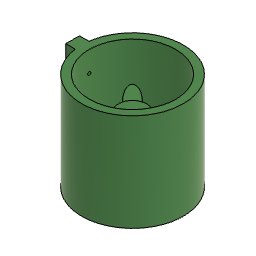
Propeller (Autodesk Fusion 360 design; units mm, degrees)
Autodesk Fusion 360 part; units mm, degrees
note: some values were not read from the file. Set by a fixed rule: which sketch regions a step uses.
sketch "Sketch1" plane through (0, 0, 0) normal (0, 0, 1) x (1, 0, 0)
  circle A0 centre (0, 0) radius 36.5
  circle A1 centre (0, 0) radius 31
  line L0 (-31, 4.9033) -> (-43, 4.9033)
  line L1 (-43, 4.9033) -> (-43, -4.9033)
  line L2 (-43, -4.9033) -> (-31, -4.9033)
  line L3 (-31, -4.9033) -> (-31, 4.9033)
  circle A2 centre (0, 0) radius 15
  line L4 (-1, 30) -> (1, 30)
  line L5 (1, 30) -> (1, 0)
  line L6 (1, 0) -> (-1, 0)
  line L7 (-1, 0) -> (-1, 30)
  line L8 (0, 0) -> (0, 30) construction
  line L9 (0, 1) -> (30, 1)
  line L10 (30, 1) -> (30, -1)
  line L11 (30, -1) -> (0, -1)
  line L12 (0, -1) -> (0, 1)
  line L13 (0, 0) -> (31, 0) construction
  line L14 (0, 0) -> (30, 0) construction
  line L15 (-43, 0) -> (-31, 0) construction
  dimension "d1" = 73
  dimension "d6" = 62
  dimension "d24" = 30
  dimension "d25" = 30
  dimension "d26" = 2
  dimension "d29" = 30
  dimension "d30" = 2
  dimension "d52" = 43
  constraint coincident A0.centre A1.centre
  constraint concentric A0 A1
  constraint horizontal L0
  constraint vertical L1
  constraint horizontal L2
  constraint vertical L3
  constraint concentric A1 A2
  constraint horizontal L4
  constraint vertical L5
  constraint horizontal L6
  constraint vertical L7
  constraint midpoint L6 A0.centre
  constraint midpoint L4 L8.end
  constraint horizontal L9
  constraint vertical L10
  constraint horizontal L11
  constraint vertical L12
  constraint coincident A1 L13.end
  constraint perpendicular L5 L13
  constraint midpoint L12 A0.centre
  constraint midpoint L10 L14.end
  constraint midpoint L1 L15.start
  constraint midpoint L3 L15.end
  constraint tangent A1 L3
  measures "d1" diameter of A0
  measures "d6" diameter of A1
  measures "d24" diameter of A2
  measures "d25" distance of L4.end L5.end
  measures "d26" distance of L5.end L6.end
  measures "d29" distance of L10.end L11.end
  measures "d30" distance of L9.end L10.end
  measures "d52" distance of A0.centre L1
extrude "Extrude3" add sketch "Sketch1" along normal blind 70 contours A0 L0 L2 L3 | A0 L0 L2 L3 | A0 L0 L1 L2 makes body 1
extrude "Extrude6" add sketch "Sketch1" along normal blind 2 separate body contours A2 L5 L6 L9 L11 L12 | A2 L9 L10 L11 | A2 L5 L9 | A2 L6 L7 L11 L12 | A2 L5 L6 L7 L9 L12 | A2 L4 L5 L7 | L5 L6 L9 L12 makes body 2
sketch "Sketch3" plane through (0, 0, 2) normal (0, 0, 1) x (-1, 0, 0)
  arc A0 (1, -14.9666) -> (-14.9666, 1) centre (0, 0) ccw
  line L0 (-14.9666, 1) -> (-30, 1)
  line L1 (-30, -1) -> (-14.9666, -1)
  arc A1 (-14.9666, -1) -> (-1, -14.9666) centre (0, 0) ccw
  line L2 (-1, -14.9666) -> (-1, -30)
  line L3 (1, -30) -> (1, -14.9666)
  circle A2 centre (0, 0) radius 15
  line L4 (0, 0) -> (-0.0958, 14.9997) construction
  line L5 (0, 0) -> (10.6066, 10.6066) construction
  line L6 (0, 0) -> (-10.6066, -10.6066) construction
  line L7 (-30, 1) -> (-30, -1)
  line L8 (-1, -30) -> (1, -30)
  constraint concentric A0 A2
  constraint coincident A0.centre A1.centre
  constraint coincident A2 L4.end
  constraint coincident A0 L4.end
  constraint midpoint A0 L5.end
  constraint midpoint A1 L6.end
extrude "Extrude7" add sketch "Sketch3" along normal blind 30 contours A0 A1 A2 bodies 2
sketch "Sketch4" plane through (0, 0, 0) normal (0, 0, 1) x (1, 0, 0)
  circle A0 centre (-80, 0) radius 10.1271
  line L0 (-80, 0) -> (-58.7868, -21.2132)
  spline S0 degree 5 poles (-80, 0) (-80.226, -0.2138) (-80.5716, -0.7482) (-80.7596, -1.8597) (-80.3329, -3.894) (-78.7401, -7.0928) (-76.249, -10.6236) (-73.0952, -14.138) (-69.5734, -17.2981) (-66.022, -19.8103) (-62.7892, -21.4385) (-60.1991, -22.0203) (-58.5181, -21.4833) (-57.9195, -19.8646) (-58.4461, -17.3315) (-60.0312, -14.1449) (-62.5165, -10.6241) (-65.6686, -7.1139) (-69.1936, -3.9501) (-72.7516, -1.4281) (-75.992, 0.2123) (-78.0688, 0.6858) (-79.2154, 0.5348) (-79.774, 0.2138) (-80, 0) knots 0 0 0 0 0 0 0.05 0.1 0.15 0.2 0.25 0.3 0.35 0.4 0.45 0.5 0.55 0.6 0.65 0.7 0.75 0.8 0.85 0.9 0.95 1 1 1 1 1 1
  line L1 (-73.1761, -13.8763) -> (-69.3934, -10.6066) construction
  line L2 (-65.5271, -7.4362) -> (-69.3934, -10.6066) construction
  line L3 (0, 0) -> (-15, 0) construction
  point P0 (-73.1761, -13.8763)
  point P1 (-65.5271, -7.4362)
  dimension "d35" = 30
  dimension "d39" = 5
  dimension "d40" = 5
  constraint coincident A0.centre L0.start
  constraint coincident P0 L1.start
  constraint midpoint L0 L1.end
  constraint coincident P1 L2.start
  constraint coincident L3.start origin
  constraint horizontal L3
  measures "d35" distance of A0.centre L0.end
  measures "d39" distance of L1.end P1
  measures "d40" distance of P0 L1.end
extrude "Extrude8" add sketch "Sketch4" along normal blind 14 separate body contours A0 S0 | A0 L0 S0 | A0 L0 S0 picked at (-77.6065, -3.8166) picked at (-76.2692, -2.3861) makes body 3
extrude "Extrude10" add sketch "Sketch4" along normal blind 10 contours A0 L0 S0 | A0 L0 S0 | A0 L0 S0 | A0 L0 S0 bodies 3
pattern_circular "C-Pattern2" count 4 over 360 about axis through (-80, 0, 14) along (0, 0, 1) of "Extrude10"
combine "Combine2" operation add target body 3 tool bodies 2 makes body 4 at (14.7847, -2.5326, 11.3333)
move_body "Move1" bodies 3 to x (1, 0, 0) y (0, 1, 0) z (0, 0, 1) at (79.8718, 0.0802, 32.4866)
combine "Combine3" operation add target body 1 tool bodies 3 4 makes body 5 at (0.5283, 3.616, 32.4866) makes body 6 at (14.7847, -2.5326, 11.3333)
sketch "Sketch6" plane through (-43, 0, 0) normal (-1, 0, 0) x (0, -1, 0)
  line L0 (-4.9033, 0) -> (4.9033, 0)
  line L1 (4.9033, 0) -> (4.9033, 70)
  line L2 (4.9033, 70) -> (-4.9033, 70)
  line L3 (-4.9033, 70) -> (-4.9033, 0)
  line L4 (-4.9033, 70) -> (4.9033, 0) construction
  line L5 (0, 35) -> (0, 15) construction
  circle A0 centre (0, 15) radius 1.15
  dimension "d57" = 20
  dimension "d58" = 2.3
  constraint coincident L2.end L3.start
  constraint coincident L0.end L1.start
  constraint midpoint L4 L5.start
  constraint perpendicular L0 L5
  constraint coincident L5.end A0.centre
  measures "d57" distance of L5.start L5.end
  measures "d58" diameter of A0
extrude "Extrude11" cut sketch "Sketch6" against normal blind 15 contours A0 bodies 1
pattern_linear "R-Pattern2" count 3 spacing 20 along (0, 0, 1) of "Extrude11"
equation "d52 = ( 72 / 2 ) * 1 mm + 7 mm"
named bodies: "Propeller", "Propeller (1)", "Propeller (2)"
